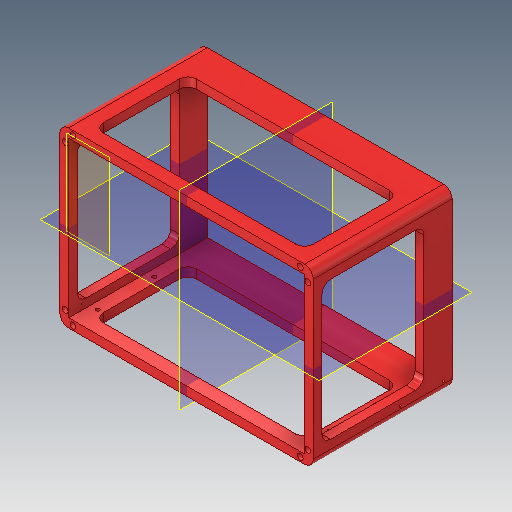
# Autodesk Inventor part: 05_Omniscope_base_v1
Saved by Autodesk Inventor 2019.4 (Build 234330000, 330)
## iProperties
Created: 2021-09-23
Part Number: 05_Omniscope_base_v1
Material: Generisch
Document SubType Name: Modeling
Designer: Muriel
Density: 1 g/cm^3
Appearance: Light Red
Author: Muriel
Autodesk Inventor part; units mm, degrees
ref_plane "Arbeitsebene1" through (0, 0, 0) normal (0, 0, 1) x (1, 0, 0)
sketch "Skizze1" plane through (0, 0, 0) normal (0, 0, 1) x (1, 0, 0)
  arc A0 (4.5124, -17.9) -> (2.1124, -17.9) centre (3.3124, -16.3) ccw construction
  line L0 (4.5124, -17.9) -> (5.3124, -17.9) construction
  line L1 (5.3124, -17.9) -> (6.3124, -16.9) construction
  line L2 (6.3124, -16.9) -> (6.3124, 16.9) construction
  line L3 (6.3124, 16.9) -> (5.3124, 17.9) construction
  line L4 (5.3124, 17.9) -> (4.5124, 17.9) construction
  arc A1 (2.1124, 17.9) -> (4.5124, 17.9) centre (3.3124, 16.3) ccw construction
  line L5 (2.1124, 17.9) -> (-7.2876, 17.9) construction
  arc A2 (-9.6876, 17.9) -> (-7.2876, 17.9) centre (-8.4876, 16.3) ccw construction
  line L6 (-9.6876, 17.9) -> (-10.4876, 17.9) construction
  line L7 (-10.4876, 17.9) -> (-11.4876, 16.9) construction
  line L8 (-11.4876, 16.9) -> (-11.4876, -16.9) construction
  line L9 (-11.4876, -16.9) -> (-10.4876, -17.9) construction
  line L10 (-10.4876, -17.9) -> (-9.6876, -17.9) construction
  arc A3 (-7.2876, -17.9) -> (-9.6876, -17.9) centre (-8.4876, -16.3) ccw construction
  line L11 (-7.2876, -17.9) -> (2.1124, -17.9) construction
  line L12 (1.5472, -2.3689) -> (1.5472, -5.8689) construction
  line L13 (1.5472, -5.8689) -> (1.0253, -5.8689) construction
  line L14 (1.0253, -5.8689) -> (-0.5233, -2.8511) construction
  line L15 (-0.5233, -2.8511) -> (-0.5233, -5.8689) construction
  line L16 (-0.5233, -5.8689) -> (-0.9572, -5.8689) construction
  line L17 (-0.9572, -5.8689) -> (-0.9572, -2.3689) construction
  line L18 (-0.9572, -2.3689) -> (-0.2964, -2.3689) construction
  line L19 (-0.2964, -2.3689) -> (1.1133, -5.14) construction
  line L20 (1.1133, -5.14) -> (1.1133, -2.3689) construction
  line L21 (1.1133, -2.3689) -> (1.5472, -2.3689) construction
  line L22 (4.5026, -1.0603) -> (4.5026, -1.4177) construction
  line L23 (4.5026, -1.4177) -> (2.7952, -1.4177) construction
  line L24 (2.7952, -1.4177) -> (2.7952, -1.0603) construction
  line L25 (2.7952, -1.0603) -> (3.4305, -1.0603) construction
  line L26 (3.4305, -1.0603) -> (3.4305, 1.2853) construction
  line L27 (3.4305, 1.2853) -> (2.7952, 1.2853) construction
  line L28 (2.7952, 1.2853) -> (2.7952, 1.6058) construction
  spline S0 degree 2 poles (2.7952, 1.6058) (3.1554, 1.6058) (3.4957, 1.81) (3.5184, 2.0937) knots 0 0 0 1 2 2 2 construction
  line L29 (3.5184, 2.0937) -> (3.8815, 2.0937) construction
  line L30 (3.8815, 2.0937) -> (3.8815, -1.0603) construction
  line L31 (3.8815, -1.0603) -> (4.5026, -1.0603) construction
  line L32 (4.5665, 6.9442) -> (5.0401, 6.9442) construction
  line L33 (5.0401, 6.9442) -> (3.8347, 3.4442) construction
  line L34 (3.8347, 3.4442) -> (3.3327, 3.4442) construction
  line L35 (3.3327, 3.4442) -> (2.1272, 6.9442) construction
  line L36 (2.1272, 6.9442) -> (2.6264, 6.9442) construction
  line L37 (2.6264, 6.9442) -> (3.5964, 4.037) construction
  line L38 (3.5964, 4.037) -> (4.5665, 6.9442) construction
  spline S1 degree 2 poles (1.5373, 5.4012) (1.7103, 5.2708) (1.8975, 4.8737) (1.8975, 4.556) knots 0 0 0 1 2 2 2 construction
  spline S2 degree 2 poles (1.8975, 4.556) (1.8975, 4.3036) (1.7358, 3.8725) (1.5883, 3.7136) knots 0 0 0 1 2 2 2 construction
  spline S3 degree 2 poles (1.5883, 3.7136) (1.4408, 3.5548) (1.0012, 3.3704) (0.7289, 3.3704) knots 0 0 0 1 2 2 2 construction
  spline S4 degree 2 poles (0.7289, 3.3704) (0.4793, 3.3704) (-0.0085, 3.4811) (-0.1872, 3.569) knots 0 0 0 1 2 2 2 construction
  line L39 (-0.1872, 3.569) -> (-0.1872, 4.0653) construction
  line L40 (-0.1872, 4.0653) -> (-0.1532, 4.0653) construction
  spline S5 degree 2 poles (-0.1532, 4.0653) (-0.0993, 4.0256) (0.1021, 3.9235) (0.2241, 3.8781) knots 0 0 0 1 2 2 2 construction
  spline S6 degree 2 poles (0.2241, 3.8781) (0.363, 3.8299) (0.5928, 3.776) (0.7374, 3.776) knots 0 0 0 1 2 2 2 construction
  spline S7 degree 2 poles (0.7374, 3.776) (0.8793, 3.776) (1.1459, 3.8781) (1.2423, 3.9888) knots 0 0 0 1 2 2 2 construction
  spline S8 degree 2 poles (1.2423, 3.9888) (1.3302, 4.0937) (1.421, 4.3717) (1.421, 4.5589) knots 0 0 0 1 2 2 2 construction
  spline S9 degree 2 poles (1.421, 4.5589) (1.421, 4.7461) (1.3189, 4.9843) (1.2224, 5.0637) knots 0 0 0 1 2 2 2 construction
  spline S10 degree 2 poles (1.2224, 5.0637) (1.1232, 5.1516) (0.8282, 5.2254) (0.6495, 5.2254) knots 0 0 0 1 2 2 2 construction
  spline S11 degree 2 poles (0.6495, 5.2254) (0.4566, 5.2254) (0.0737, 5.1658) (-0.0425, 5.1403) knots 0 0 0 1 2 2 2 construction
  line L41 (-0.0425, 5.1403) -> (-0.0425, 6.9442) construction
  line L42 (-0.0425, 6.9442) -> (1.8776, 6.9442) construction
  line L43 (1.8776, 6.9442) -> (1.8776, 6.5329) construction
  line L44 (1.8776, 6.5329) -> (0.4084, 6.5329) construction
  line L45 (0.4084, 6.5329) -> (0.4084, 5.5998) construction
  spline S12 degree 2 poles (0.4084, 5.5998) (0.4935, 5.6111) (0.658, 5.6196) (0.7261, 5.6196) knots 0 0 0 1 2 2 2 construction
  spline S13 degree 2 poles (0.7261, 5.6196) (0.9955, 5.6196) (1.3671, 5.5317) (1.5373, 5.4012) knots 0 0 0 1 2 2 2 construction
  line L46 (1.0905, -1.4177) -> (0.6254, -1.4177) construction
  line L47 (0.6254, -1.4177) -> (0.6254, 1.6682) construction
  line L48 (0.6254, 1.6682) -> (-0.5488, 1.6682) construction
  line L49 (-0.5488, 1.6682) -> (-0.5488, 2.0823) construction
  line L50 (-0.5488, 2.0823) -> (2.2648, 2.0823) construction
  line L51 (2.2648, 2.0823) -> (2.2648, 1.6682) construction
  line L52 (2.2648, 1.6682) -> (1.0905, 1.6682) construction
  line L53 (1.0905, 1.6682) -> (1.0905, -1.4177) construction
  spline S14 degree 2 poles (-2.0577, -5.8349) (-2.2307, -5.886) (-2.5087, -5.937) (-2.7044, -5.937) knots 0 0 0 1 2 2 2 construction
  spline S15 degree 2 poles (-2.7044, -5.937) (-3.076, -5.937) (-3.6914, -5.7101) (-3.9127, -5.4804) knots 0 0 0 1 2 2 2 construction
  spline S16 degree 2 poles (-3.9127, -5.4804) (-4.1339, -5.2478) (-4.3693, -4.5614) (-4.3693, -4.1161) knots 0 0 0 1 2 2 2 construction
  spline S17 degree 2 poles (-4.3693, -4.1161) (-4.3693, -3.6935) (-4.1311, -3.0241) (-3.9098, -2.7859) knots 0 0 0 1 2 2 2 construction
  spline S18 degree 2 poles (-3.9098, -2.7859) (-3.6971, -2.5561) (-3.0731, -2.3065) (-2.7016, -2.3065) knots 0 0 0 1 2 2 2 construction
  spline S19 degree 2 poles (-2.7016, -2.3065) (-2.5229, -2.3065) (-2.1995, -2.3576) (-2.052, -2.403) knots 0 0 0 1 2 2 2 construction
  spline S20 degree 2 poles (-2.052, -2.403) (-1.9329, -2.437) (-1.6436, -2.5618) (-1.5557, -2.6072) knots 0 0 0 1 2 2 2 construction
  line L54 (-1.5557, -2.6072) -> (-1.5557, -3.1688) construction
  line L55 (-1.5557, -3.1688) -> (-1.5954, -3.1688) construction
  spline S21 degree 2 poles (-1.5954, -3.1688) (-1.6833, -3.0922) (-1.8677, -2.9532) (-2.0379, -2.8738) knots 0 0 0 1 2 2 2 construction
  spline S22 degree 2 poles (-2.0379, -2.8738) (-2.1797, -2.8029) (-2.5456, -2.7093) (-2.7554, -2.7093) knots 0 0 0 1 2 2 2 construction
  spline S23 degree 2 poles (-2.7554, -2.7093) (-3.2603, -2.7093) (-3.8843, -3.4694) (-3.8843, -4.1019) knots 0 0 0 1 2 2 2 construction
  spline S24 degree 2 poles (-3.8843, -4.1019) (-3.8843, -4.4536) (-3.7198, -4.9812) (-3.5638, -5.1627) knots 0 0 0 1 2 2 2 construction
  spline S25 degree 2 poles (-3.5638, -5.1627) (-3.4135, -5.3442) (-2.988, -5.5343) (-2.7214, -5.5343) knots 0 0 0 1 2 2 2 construction
  spline S26 degree 2 poles (-2.7214, -5.5343) (-2.5257, -5.5343) (-2.1343, -5.4775) (-2.001, -5.4208) knots 0 0 0 1 2 2 2 construction
  line L56 (-2.001, -5.4208) -> (-2.001, -4.516) construction
  line L57 (-2.001, -4.516) -> (-2.8122, -4.516) construction
  line L58 (-2.8122, -4.516) -> (-2.8122, -4.1076) construction
  line L59 (-2.8122, -4.1076) -> (-1.5415, -4.1076) construction
  line L60 (-1.5415, -4.1076) -> (-1.5415, -5.6364) construction
  spline S27 degree 2 poles (-1.5415, -5.6364) (-1.6294, -5.6761) (-1.9301, -5.798) (-2.0577, -5.8349) knots 0 0 0 1 2 2 2 construction
  spline S28 degree 2 poles (4.307, -2.6469) (4.6445, -2.871) (5.016, -3.6112) (5.016, -4.1218) knots 0 0 0 1 2 2 2 construction
  spline S29 degree 2 poles (5.016, -4.1218) (5.016, -4.6011) (4.6275, -5.3726) (4.3013, -5.5881) knots 0 0 0 1 2 2 2 construction
  spline S30 degree 2 poles (4.3013, -5.5881) (4.0347, -5.7555) (3.4873, -5.8689) (3.0618, -5.8689) knots 0 0 0 1 2 2 2 construction
  line L61 (3.0618, -5.8689) -> (2.2563, -5.8689) construction
  line L62 (2.2563, -5.8689) -> (2.2563, -2.3689) construction
  line L63 (2.2563, -2.3689) -> (3.0533, -2.3689) construction
  spline S31 degree 2 poles (3.0533, -2.3689) (3.5468, -2.3689) (4.1084, -2.5164) (4.307, -2.6469) knots 0 0 0 1 2 2 2 construction
  arc A4 (4.5124, -53.9) -> (2.1124, -53.9) centre (3.3124, -52.3) ccw construction
  line L64 (4.5124, -53.9) -> (5.3124, -53.9) construction
  line L65 (5.3124, -53.9) -> (6.3124, -52.9) construction
  line L66 (6.3124, -52.9) -> (6.3124, -19.1) construction
  line L67 (6.3124, -19.1) -> (5.3124, -18.1) construction
  line L68 (5.3124, -18.1) -> (4.5124, -18.1) construction
  arc A5 (2.1124, -18.1) -> (4.5124, -18.1) centre (3.3124, -19.7) ccw construction
  line L69 (2.1124, -18.1) -> (-7.2876, -18.1) construction
  arc A6 (-9.6876, -18.1) -> (-7.2876, -18.1) centre (-8.4876, -19.7) ccw construction
  line L70 (-9.6876, -18.1) -> (-10.4876, -18.1) construction
  line L71 (-10.4876, -18.1) -> (-11.4876, -19.1) construction
  line L72 (-11.4876, -19.1) -> (-11.4876, -52.9) construction
  line L73 (-11.4876, -52.9) -> (-10.4876, -53.9) construction
  line L74 (-10.4876, -53.9) -> (-9.6876, -53.9) construction
  arc A7 (-7.2876, -53.9) -> (-9.6876, -53.9) centre (-8.4876, -52.3) ccw construction
  line L75 (-7.2876, -53.9) -> (2.1124, -53.9) construction
  line L76 (1.5472, -38.3689) -> (1.5472, -41.8689) construction
  line L77 (1.5472, -41.8689) -> (1.0253, -41.8689) construction
  line L78 (1.0253, -41.8689) -> (-0.5233, -38.8511) construction
  line L79 (-0.5233, -38.8511) -> (-0.5233, -41.8689) construction
  line L80 (-0.5233, -41.8689) -> (-0.9572, -41.8689) construction
  line L81 (-0.9572, -41.8689) -> (-0.9572, -38.3689) construction
  line L82 (-0.9572, -38.3689) -> (-0.2964, -38.3689) construction
  line L83 (-0.2964, -38.3689) -> (1.1133, -41.14) construction
  line L84 (1.1133, -41.14) -> (1.1133, -38.3689) construction
  line L85 (1.1133, -38.3689) -> (1.5472, -38.3689) construction
  line L86 (4.5026, -37.0603) -> (4.5026, -37.4177) construction
  line L87 (4.5026, -37.4177) -> (2.7952, -37.4177) construction
  line L88 (2.7952, -37.4177) -> (2.7952, -37.0603) construction
  line L89 (2.7952, -37.0603) -> (3.4305, -37.0603) construction
  line L90 (3.4305, -37.0603) -> (3.4305, -34.7147) construction
  line L91 (3.4305, -34.7147) -> (2.7952, -34.7147) construction
  line L92 (2.7952, -34.7147) -> (2.7952, -34.3942) construction
  spline S32 degree 2 poles (2.7952, -34.3942) (3.1554, -34.3942) (3.4957, -34.19) (3.5184, -33.9063) knots 0 0 0 1 2 2 2 construction
  line L93 (3.5184, -33.9063) -> (3.8815, -33.9063) construction
  line L94 (3.8815, -33.9063) -> (3.8815, -37.0603) construction
  line L95 (3.8815, -37.0603) -> (4.5026, -37.0603) construction
  line L96 (4.5665, -29.0558) -> (5.0401, -29.0558) construction
  line L97 (5.0401, -29.0558) -> (3.8347, -32.5558) construction
  line L98 (3.8347, -32.5558) -> (3.3327, -32.5558) construction
  line L99 (3.3327, -32.5558) -> (2.1272, -29.0558) construction
  line L100 (2.1272, -29.0558) -> (2.6264, -29.0558) construction
  line L101 (2.6264, -29.0558) -> (3.5964, -31.963) construction
  line L102 (3.5964, -31.963) -> (4.5665, -29.0558) construction
  spline S33 degree 2 poles (1.5373, -30.5988) (1.7103, -30.7292) (1.8975, -31.1263) (1.8975, -31.444) knots 0 0 0 1 2 2 2 construction
  spline S34 degree 2 poles (1.8975, -31.444) (1.8975, -31.6964) (1.7358, -32.1275) (1.5883, -32.2864) knots 0 0 0 1 2 2 2 construction
  spline S35 degree 2 poles (1.5883, -32.2864) (1.4408, -32.4452) (1.0012, -32.6296) (0.7289, -32.6296) knots 0 0 0 1 2 2 2 construction
  spline S36 degree 2 poles (0.7289, -32.6296) (0.4793, -32.6296) (-0.0085, -32.5189) (-0.1872, -32.431) knots 0 0 0 1 2 2 2 construction
  line L103 (-0.1872, -32.431) -> (-0.1872, -31.9347) construction
  line L104 (-0.1872, -31.9347) -> (-0.1532, -31.9347) construction
  spline S37 degree 2 poles (-0.1532, -31.9347) (-0.0993, -31.9744) (0.1021, -32.0765) (0.2241, -32.1219) knots 0 0 0 1 2 2 2 construction
  spline S38 degree 2 poles (0.2241, -32.1219) (0.363, -32.1701) (0.5928, -32.224) (0.7374, -32.224) knots 0 0 0 1 2 2 2 construction
  spline S39 degree 2 poles (0.7374, -32.224) (0.8793, -32.224) (1.1459, -32.1219) (1.2423, -32.0112) knots 0 0 0 1 2 2 2 construction
  spline S40 degree 2 poles (1.2423, -32.0112) (1.3302, -31.9063) (1.421, -31.6283) (1.421, -31.4411) knots 0 0 0 1 2 2 2 construction
  spline S41 degree 2 poles (1.421, -31.4411) (1.421, -31.2539) (1.3189, -31.0157) (1.2224, -30.9363) knots 0 0 0 1 2 2 2 construction
  spline S42 degree 2 poles (1.2224, -30.9363) (1.1232, -30.8484) (0.8282, -30.7746) (0.6495, -30.7746) knots 0 0 0 1 2 2 2 construction
  spline S43 degree 2 poles (0.6495, -30.7746) (0.4566, -30.7746) (0.0737, -30.8342) (-0.0425, -30.8597) knots 0 0 0 1 2 2 2 construction
  line L105 (-0.0425, -30.8597) -> (-0.0425, -29.0558) construction
  line L106 (-0.0425, -29.0558) -> (1.8776, -29.0558) construction
  line L107 (1.8776, -29.0558) -> (1.8776, -29.4671) construction
  line L108 (1.8776, -29.4671) -> (0.4084, -29.4671) construction
  line L109 (0.4084, -29.4671) -> (0.4084, -30.4002) construction
  spline S44 degree 2 poles (0.4084, -30.4002) (0.4935, -30.3889) (0.658, -30.3804) (0.7261, -30.3804) knots 0 0 0 1 2 2 2 construction
  spline S45 degree 2 poles (0.7261, -30.3804) (0.9955, -30.3804) (1.3671, -30.4683) (1.5373, -30.5988) knots 0 0 0 1 2 2 2 construction
  line L110 (1.0905, -37.4177) -> (0.6254, -37.4177) construction
  line L111 (0.6254, -37.4177) -> (0.6254, -34.3318) construction
  line L112 (0.6254, -34.3318) -> (-0.5488, -34.3318) construction
  line L113 (-0.5488, -34.3318) -> (-0.5488, -33.9177) construction
  line L114 (-0.5488, -33.9177) -> (2.2648, -33.9177) construction
  line L115 (2.2648, -33.9177) -> (2.2648, -34.3318) construction
  line L116 (2.2648, -34.3318) -> (1.0905, -34.3318) construction
  line L117 (1.0905, -34.3318) -> (1.0905, -37.4177) construction
  spline S46 degree 2 poles (-2.0577, -41.8349) (-2.2307, -41.886) (-2.5087, -41.937) (-2.7044, -41.937) knots 0 0 0 1 2 2 2 construction
  spline S47 degree 2 poles (-2.7044, -41.937) (-3.076, -41.937) (-3.6914, -41.7101) (-3.9127, -41.4804) knots 0 0 0 1 2 2 2 construction
  spline S48 degree 2 poles (-3.9127, -41.4804) (-4.1339, -41.2478) (-4.3693, -40.5614) (-4.3693, -40.1161) knots 0 0 0 1 2 2 2 construction
  spline S49 degree 2 poles (-4.3693, -40.1161) (-4.3693, -39.6935) (-4.1311, -39.0241) (-3.9098, -38.7859) knots 0 0 0 1 2 2 2 construction
  spline S50 degree 2 poles (-3.9098, -38.7859) (-3.6971, -38.5561) (-3.0731, -38.3065) (-2.7016, -38.3065) knots 0 0 0 1 2 2 2 construction
  spline S51 degree 2 poles (-2.7016, -38.3065) (-2.5229, -38.3065) (-2.1995, -38.3576) (-2.052, -38.403) knots 0 0 0 1 2 2 2 construction
  spline S52 degree 2 poles (-2.052, -38.403) (-1.9329, -38.437) (-1.6436, -38.5618) (-1.5557, -38.6072) knots 0 0 0 1 2 2 2 construction
  line L118 (-1.5557, -38.6072) -> (-1.5557, -39.1688) construction
  line L119 (-1.5557, -39.1688) -> (-1.5954, -39.1688) construction
  spline S53 degree 2 poles (-1.5954, -39.1688) (-1.6833, -39.0922) (-1.8677, -38.9532) (-2.0379, -38.8738) knots 0 0 0 1 2 2 2 construction
  spline S54 degree 2 poles (-2.0379, -38.8738) (-2.1797, -38.8029) (-2.5456, -38.7093) (-2.7554, -38.7093) knots 0 0 0 1 2 2 2 construction
  spline S55 degree 2 poles (-2.7554, -38.7093) (-3.2603, -38.7093) (-3.8843, -39.4694) (-3.8843, -40.1019) knots 0 0 0 1 2 2 2 construction
  spline S56 degree 2 poles (-3.8843, -40.1019) (-3.8843, -40.4536) (-3.7198, -40.9812) (-3.5638, -41.1627) knots 0 0 0 1 2 2 2 construction
  spline S57 degree 2 poles (-3.5638, -41.1627) (-3.4135, -41.3442) (-2.988, -41.5343) (-2.7214, -41.5343) knots 0 0 0 1 2 2 2 construction
  spline S58 degree 2 poles (-2.7214, -41.5343) (-2.5257, -41.5343) (-2.1343, -41.4775) (-2.001, -41.4208) knots 0 0 0 1 2 2 2 construction
  line L120 (-2.001, -41.4208) -> (-2.001, -40.516) construction
  line L121 (-2.001, -40.516) -> (-2.8122, -40.516) construction
  line L122 (-2.8122, -40.516) -> (-2.8122, -40.1076) construction
  line L123 (-2.8122, -40.1076) -> (-1.5415, -40.1076) construction
  line L124 (-1.5415, -40.1076) -> (-1.5415, -41.6364) construction
  spline S59 degree 2 poles (-1.5415, -41.6364) (-1.6294, -41.6761) (-1.9301, -41.798) (-2.0577, -41.8349) knots 0 0 0 1 2 2 2 construction
  spline S60 degree 2 poles (4.307, -38.6469) (4.6445, -38.871) (5.016, -39.6112) (5.016, -40.1218) knots 0 0 0 1 2 2 2 construction
  spline S61 degree 2 poles (5.016, -40.1218) (5.016, -40.6011) (4.6275, -41.3726) (4.3013, -41.5881) knots 0 0 0 1 2 2 2 construction
  spline S62 degree 2 poles (4.3013, -41.5881) (4.0347, -41.7555) (3.4873, -41.8689) (3.0618, -41.8689) knots 0 0 0 1 2 2 2 construction
  line L125 (3.0618, -41.8689) -> (2.2563, -41.8689) construction
  line L126 (2.2563, -41.8689) -> (2.2563, -38.3689) construction
  line L127 (2.2563, -38.3689) -> (3.0533, -38.3689) construction
  spline S63 degree 2 poles (3.0533, -38.3689) (3.5468, -38.3689) (4.1084, -38.5164) (4.307, -38.6469) knots 0 0 0 1 2 2 2 construction
  arc A8 (94.5124, -53.9) -> (92.1124, -53.9) centre (93.3124, -52.3) ccw construction
  line L128 (94.5124, -53.9) -> (95.3124, -53.9) construction
  line L129 (95.3124, -53.9) -> (96.3124, -52.9) construction
  line L130 (96.3124, -52.9) -> (96.3124, -19.1) construction
  line L131 (96.3124, -19.1) -> (95.3124, -18.1) construction
  line L132 (95.3124, -18.1) -> (94.5124, -18.1) construction
  arc A9 (92.1124, -18.1) -> (94.5124, -18.1) centre (93.3124, -19.7) ccw construction
  line L133 (92.1124, -18.1) -> (82.7124, -18.1) construction
  arc A10 (80.3124, -18.1) -> (82.7124, -18.1) centre (81.5124, -19.7) ccw construction
  line L134 (80.3124, -18.1) -> (79.5124, -18.1) construction
  line L135 (79.5124, -18.1) -> (78.5124, -19.1) construction
  line L136 (78.5124, -19.1) -> (78.5124, -52.9) construction
  line L137 (78.5124, -52.9) -> (79.5124, -53.9) construction
  line L138 (79.5124, -53.9) -> (80.3124, -53.9) construction
  arc A11 (82.7124, -53.9) -> (80.3124, -53.9) centre (81.5124, -52.3) ccw construction
  line L139 (82.7124, -53.9) -> (92.1124, -53.9) construction
  line L140 (91.5472, -38.3689) -> (91.5472, -41.8689) construction
  line L141 (91.5472, -41.8689) -> (91.0253, -41.8689) construction
  line L142 (91.0253, -41.8689) -> (89.4767, -38.8511) construction
  line L143 (89.4767, -38.8511) -> (89.4767, -41.8689) construction
  line L144 (89.4767, -41.8689) -> (89.0428, -41.8689) construction
  line L145 (89.0428, -41.8689) -> (89.0428, -38.3689) construction
  line L146 (89.0428, -38.3689) -> (89.7036, -38.3689) construction
  line L147 (89.7036, -38.3689) -> (91.1133, -41.14) construction
  line L148 (91.1133, -41.14) -> (91.1133, -38.3689) construction
  line L149 (91.1133, -38.3689) -> (91.5472, -38.3689) construction
  line L150 (94.5026, -37.0603) -> (94.5026, -37.4177) construction
  line L151 (94.5026, -37.4177) -> (92.7952, -37.4177) construction
  line L152 (92.7952, -37.4177) -> (92.7952, -37.0603) construction
  line L153 (92.7952, -37.0603) -> (93.4305, -37.0603) construction
  line L154 (93.4305, -37.0603) -> (93.4305, -34.7147) construction
  line L155 (93.4305, -34.7147) -> (92.7952, -34.7147) construction
  line L156 (92.7952, -34.7147) -> (92.7952, -34.3942) construction
  spline S64 degree 2 poles (92.7952, -34.3942) (93.1554, -34.3942) (93.4957, -34.19) (93.5184, -33.9063) knots 0 0 0 1 2 2 2 construction
  line L157 (93.5184, -33.9063) -> (93.8815, -33.9063) construction
  line L158 (93.8815, -33.9063) -> (93.8815, -37.0603) construction
  line L159 (93.8815, -37.0603) -> (94.5026, -37.0603) construction
  line L160 (94.5665, -29.0558) -> (95.0401, -29.0558) construction
  line L161 (95.0401, -29.0558) -> (93.8347, -32.5558) construction
  line L162 (93.8347, -32.5558) -> (93.3327, -32.5558) construction
  line L163 (93.3327, -32.5558) -> (92.1272, -29.0558) construction
  line L164 (92.1272, -29.0558) -> (92.6264, -29.0558) construction
  line L165 (92.6264, -29.0558) -> (93.5964, -31.963) construction
  line L166 (93.5964, -31.963) -> (94.5665, -29.0558) construction
  spline S65 degree 2 poles (91.5373, -30.5988) (91.7103, -30.7292) (91.8975, -31.1263) (91.8975, -31.444) knots 0 0 0 1 2 2 2 construction
  spline S66 degree 2 poles (91.8975, -31.444) (91.8975, -31.6964) (91.7358, -32.1275) (91.5883, -32.2864) knots 0 0 0 1 2 2 2 construction
  spline S67 degree 2 poles (91.5883, -32.2864) (91.4408, -32.4452) (91.0012, -32.6296) (90.7289, -32.6296) knots 0 0 0 1 2 2 2 construction
  spline S68 degree 2 poles (90.7289, -32.6296) (90.4793, -32.6296) (89.9915, -32.5189) (89.8128, -32.431) knots 0 0 0 1 2 2 2 construction
  line L167 (89.8128, -32.431) -> (89.8128, -31.9347) construction
  line L168 (89.8128, -31.9347) -> (89.8468, -31.9347) construction
  spline S69 degree 2 poles (89.8468, -31.9347) (89.9007, -31.9744) (90.1021, -32.0765) (90.2241, -32.1219) knots 0 0 0 1 2 2 2 construction
  spline S70 degree 2 poles (90.2241, -32.1219) (90.363, -32.1701) (90.5928, -32.224) (90.7374, -32.224) knots 0 0 0 1 2 2 2 construction
  spline S71 degree 2 poles (90.7374, -32.224) (90.8793, -32.224) (91.1459, -32.1219) (91.2423, -32.0112) knots 0 0 0 1 2 2 2 construction
  spline S72 degree 2 poles (91.2423, -32.0112) (91.3302, -31.9063) (91.421, -31.6283) (91.421, -31.4411) knots 0 0 0 1 2 2 2 construction
  spline S73 degree 2 poles (91.421, -31.4411) (91.421, -31.2539) (91.3189, -31.0157) (91.2224, -30.9363) knots 0 0 0 1 2 2 2 construction
  spline S74 degree 2 poles (91.2224, -30.9363) (91.1232, -30.8484) (90.8282, -30.7746) (90.6495, -30.7746) knots 0 0 0 1 2 2 2 construction
  spline S75 degree 2 poles (90.6495, -30.7746) (90.4566, -30.7746) (90.0737, -30.8342) (89.9575, -30.8597) knots 0 0 0 1 2 2 2 construction
  line L169 (89.9575, -30.8597) -> (89.9575, -29.0558) construction
  line L170 (89.9575, -29.0558) -> (91.8776, -29.0558) construction
  line L171 (91.8776, -29.0558) -> (91.8776, -29.4671) construction
  line L172 (91.8776, -29.4671) -> (90.4084, -29.4671) construction
  line L173 (90.4084, -29.4671) -> (90.4084, -30.4002) construction
  spline S76 degree 2 poles (90.4084, -30.4002) (90.4935, -30.3889) (90.658, -30.3804) (90.7261, -30.3804) knots 0 0 0 1 2 2 2 construction
  spline S77 degree 2 poles (90.7261, -30.3804) (90.9955, -30.3804) (91.3671, -30.4683) (91.5373, -30.5988) knots 0 0 0 1 2 2 2 construction
  line L174 (91.0905, -37.4177) -> (90.6254, -37.4177) construction
  line L175 (90.6254, -37.4177) -> (90.6254, -34.3318) construction
  line L176 (90.6254, -34.3318) -> (89.4512, -34.3318) construction
  line L177 (89.4512, -34.3318) -> (89.4512, -33.9177) construction
  line L178 (89.4512, -33.9177) -> (92.2648, -33.9177) construction
  line L179 (92.2648, -33.9177) -> (92.2648, -34.3318) construction
  line L180 (92.2648, -34.3318) -> (91.0905, -34.3318) construction
  line L181 (91.0905, -34.3318) -> (91.0905, -37.4177) construction
  spline S78 degree 2 poles (87.9423, -41.8349) (87.7693, -41.886) (87.4913, -41.937) (87.2956, -41.937) knots 0 0 0 1 2 2 2 construction
  spline S79 degree 2 poles (87.2956, -41.937) (86.924, -41.937) (86.3086, -41.7101) (86.0873, -41.4804) knots 0 0 0 1 2 2 2 construction
  spline S80 degree 2 poles (86.0873, -41.4804) (85.8661, -41.2478) (85.6307, -40.5614) (85.6307, -40.1161) knots 0 0 0 1 2 2 2 construction
  spline S81 degree 2 poles (85.6307, -40.1161) (85.6307, -39.6935) (85.8689, -39.0241) (86.0902, -38.7859) knots 0 0 0 1 2 2 2 construction
  spline S82 degree 2 poles (86.0902, -38.7859) (86.3029, -38.5561) (86.9269, -38.3065) (87.2984, -38.3065) knots 0 0 0 1 2 2 2 construction
  spline S83 degree 2 poles (87.2984, -38.3065) (87.4771, -38.3065) (87.8005, -38.3576) (87.948, -38.403) knots 0 0 0 1 2 2 2 construction
  spline S84 degree 2 poles (87.948, -38.403) (88.0671, -38.437) (88.3564, -38.5618) (88.4443, -38.6072) knots 0 0 0 1 2 2 2 construction
  line L182 (88.4443, -38.6072) -> (88.4443, -39.1688) construction
  line L183 (88.4443, -39.1688) -> (88.4046, -39.1688) construction
  spline S85 degree 2 poles (88.4046, -39.1688) (88.3167, -39.0922) (88.1323, -38.9532) (87.9621, -38.8738) knots 0 0 0 1 2 2 2 construction
  spline S86 degree 2 poles (87.9621, -38.8738) (87.8203, -38.8029) (87.4544, -38.7093) (87.2446, -38.7093) knots 0 0 0 1 2 2 2 construction
  spline S87 degree 2 poles (87.2446, -38.7093) (86.7397, -38.7093) (86.1157, -39.4694) (86.1157, -40.1019) knots 0 0 0 1 2 2 2 construction
  spline S88 degree 2 poles (86.1157, -40.1019) (86.1157, -40.4536) (86.2802, -40.9812) (86.4362, -41.1627) knots 0 0 0 1 2 2 2 construction
  spline S89 degree 2 poles (86.4362, -41.1627) (86.5865, -41.3442) (87.012, -41.5343) (87.2786, -41.5343) knots 0 0 0 1 2 2 2 construction
  spline S90 degree 2 poles (87.2786, -41.5343) (87.4743, -41.5343) (87.8657, -41.4775) (87.999, -41.4208) knots 0 0 0 1 2 2 2 construction
  line L184 (87.999, -41.4208) -> (87.999, -40.516) construction
  line L185 (87.999, -40.516) -> (87.1878, -40.516) construction
  line L186 (87.1878, -40.516) -> (87.1878, -40.1076) construction
  line L187 (87.1878, -40.1076) -> (88.4585, -40.1076) construction
  line L188 (88.4585, -40.1076) -> (88.4585, -41.6364) construction
  spline S91 degree 2 poles (88.4585, -41.6364) (88.3706, -41.6761) (88.0699, -41.798) (87.9423, -41.8349) knots 0 0 0 1 2 2 2 construction
  spline S92 degree 2 poles (94.307, -38.6469) (94.6445, -38.871) (95.016, -39.6112) (95.016, -40.1218) knots 0 0 0 1 2 2 2 construction
  spline S93 degree 2 poles (95.016, -40.1218) (95.016, -40.6011) (94.6275, -41.3726) (94.3013, -41.5881) knots 0 0 0 1 2 2 2 construction
  spline S94 degree 2 poles (94.3013, -41.5881) (94.0347, -41.7555) (93.4873, -41.8689) (93.0618, -41.8689) knots 0 0 0 1 2 2 2 construction
  line L189 (93.0618, -41.8689) -> (92.2563, -41.8689) construction
  line L190 (92.2563, -41.8689) -> (92.2563, -38.3689) construction
  line L191 (92.2563, -38.3689) -> (93.0533, -38.3689) construction
  spline S95 degree 2 poles (93.0533, -38.3689) (93.5468, -38.3689) (94.1084, -38.5164) (94.307, -38.6469) knots 0 0 0 1 2 2 2 construction
  arc A12 (94.5124, -17.9) -> (92.1124, -17.9) centre (93.3124, -16.3) ccw construction
  line L192 (94.5124, -17.9) -> (95.3124, -17.9) construction
  line L193 (95.3124, -17.9) -> (96.3124, -16.9) construction
  line L194 (96.3124, -16.9) -> (96.3124, 16.9) construction
  line L195 (96.3124, 16.9) -> (95.3124, 17.9) construction
  line L196 (95.3124, 17.9) -> (94.5124, 17.9) construction
  arc A13 (92.1124, 17.9) -> (94.5124, 17.9) centre (93.3124, 16.3) ccw construction
  line L197 (92.1124, 17.9) -> (82.7124, 17.9) construction
  arc A14 (80.3124, 17.9) -> (82.7124, 17.9) centre (81.5124, 16.3) ccw construction
  line L198 (80.3124, 17.9) -> (79.5124, 17.9) construction
  line L199 (79.5124, 17.9) -> (78.5124, 16.9) construction
  line L200 (78.5124, 16.9) -> (78.5124, -16.9) construction
  line L201 (78.5124, -16.9) -> (79.5124, -17.9) construction
  line L202 (79.5124, -17.9) -> (80.3124, -17.9) construction
  arc A15 (82.7124, -17.9) -> (80.3124, -17.9) centre (81.5124, -16.3) ccw construction
  line L203 (82.7124, -17.9) -> (92.1124, -17.9) construction
  line L204 (91.5472, -2.3689) -> (91.5472, -5.8689) construction
  line L205 (91.5472, -5.8689) -> (91.0253, -5.8689) construction
  line L206 (91.0253, -5.8689) -> (89.4767, -2.8511) construction
  line L207 (89.4767, -2.8511) -> (89.4767, -5.8689) construction
  line L208 (89.4767, -5.8689) -> (89.0428, -5.8689) construction
  line L209 (89.0428, -5.8689) -> (89.0428, -2.3689) construction
  line L210 (89.0428, -2.3689) -> (89.7036, -2.3689) construction
  line L211 (89.7036, -2.3689) -> (91.1133, -5.14) construction
  line L212 (91.1133, -5.14) -> (91.1133, -2.3689) construction
  line L213 (91.1133, -2.3689) -> (91.5472, -2.3689) construction
  line L214 (94.5026, -1.0603) -> (94.5026, -1.4177) construction
  line L215 (94.5026, -1.4177) -> (92.7952, -1.4177) construction
  line L216 (92.7952, -1.4177) -> (92.7952, -1.0603) construction
  line L217 (92.7952, -1.0603) -> (93.4305, -1.0603) construction
  line L218 (93.4305, -1.0603) -> (93.4305, 1.2853) construction
  line L219 (93.4305, 1.2853) -> (92.7952, 1.2853) construction
  line L220 (92.7952, 1.2853) -> (92.7952, 1.6058) construction
  spline S96 degree 2 poles (92.7952, 1.6058) (93.1554, 1.6058) (93.4957, 1.81) (93.5184, 2.0937) knots 0 0 0 1 2 2 2 construction
  line L221 (93.5184, 2.0937) -> (93.8815, 2.0937) construction
  line L222 (93.8815, 2.0937) -> (93.8815, -1.0603) construction
  line L223 (93.8815, -1.0603) -> (94.5026, -1.0603) construction
  line L224 (94.5665, 6.9442) -> (95.0401, 6.9442) construction
  line L225 (95.0401, 6.9442) -> (93.8347, 3.4442) construction
  line L226 (93.8347, 3.4442) -> (93.3327, 3.4442) construction
  line L227 (93.3327, 3.4442) -> (92.1272, 6.9442) construction
  line L228 (92.1272, 6.9442) -> (92.6264, 6.9442) construction
  line L229 (92.6264, 6.9442) -> (93.5964, 4.037) construction
  line L230 (93.5964, 4.037) -> (94.5665, 6.9442) construction
  spline S97 degree 2 poles (91.5373, 5.4012) (91.7103, 5.2708) (91.8975, 4.8737) (91.8975, 4.556) knots 0 0 0 1 2 2 2 construction
  spline S98 degree 2 poles (91.8975, 4.556) (91.8975, 4.3036) (91.7358, 3.8725) (91.5883, 3.7136) knots 0 0 0 1 2 2 2 construction
  spline S99 degree 2 poles (91.5883, 3.7136) (91.4408, 3.5548) (91.0012, 3.3704) (90.7289, 3.3704) knots 0 0 0 1 2 2 2 construction
  spline S100 degree 2 poles (90.7289, 3.3704) (90.4793, 3.3704) (89.9915, 3.4811) (89.8128, 3.569) knots 0 0 0 1 2 2 2 construction
  line L231 (89.8128, 3.569) -> (89.8128, 4.0653) construction
  line L232 (89.8128, 4.0653) -> (89.8468, 4.0653) construction
  spline S101 degree 2 poles (89.8468, 4.0653) (89.9007, 4.0256) (90.1021, 3.9235) (90.2241, 3.8781) knots 0 0 0 1 2 2 2 construction
  spline S102 degree 2 poles (90.2241, 3.8781) (90.363, 3.8299) (90.5928, 3.776) (90.7374, 3.776) knots 0 0 0 1 2 2 2 construction
  spline S103 degree 2 poles (90.7374, 3.776) (90.8793, 3.776) (91.1459, 3.8781) (91.2423, 3.9888) knots 0 0 0 1 2 2 2 construction
  spline S104 degree 2 poles (91.2423, 3.9888) (91.3302, 4.0937) (91.421, 4.3717) (91.421, 4.5589) knots 0 0 0 1 2 2 2 construction
  spline S105 degree 2 poles (91.421, 4.5589) (91.421, 4.7461) (91.3189, 4.9843) (91.2224, 5.0637) knots 0 0 0 1 2 2 2 construction
  spline S106 degree 2 poles (91.2224, 5.0637) (91.1232, 5.1516) (90.8282, 5.2254) (90.6495, 5.2254) knots 0 0 0 1 2 2 2 construction
  spline S107 degree 2 poles (90.6495, 5.2254) (90.4566, 5.2254) (90.0737, 5.1658) (89.9575, 5.1403) knots 0 0 0 1 2 2 2 construction
  line L233 (89.9575, 5.1403) -> (89.9575, 6.9442) construction
  line L234 (89.9575, 6.9442) -> (91.8776, 6.9442) construction
  line L235 (91.8776, 6.9442) -> (91.8776, 6.5329) construction
  line L236 (91.8776, 6.5329) -> (90.4084, 6.5329) construction
  line L237 (90.4084, 6.5329) -> (90.4084, 5.5998) construction
  spline S108 degree 2 poles (90.4084, 5.5998) (90.4935, 5.6111) (90.658, 5.6196) (90.7261, 5.6196) knots 0 0 0 1 2 2 2 construction
  spline S109 degree 2 poles (90.7261, 5.6196) (90.9955, 5.6196) (91.3671, 5.5317) (91.5373, 5.4012) knots 0 0 0 1 2 2 2 construction
  line L238 (91.0905, -1.4177) -> (90.6254, -1.4177) construction
  line L239 (90.6254, -1.4177) -> (90.6254, 1.6682) construction
  line L240 (90.6254, 1.6682) -> (89.4512, 1.6682) construction
  line L241 (89.4512, 1.6682) -> (89.4512, 2.0823) construction
  line L242 (89.4512, 2.0823) -> (92.2648, 2.0823) construction
  line L243 (92.2648, 2.0823) -> (92.2648, 1.6682) construction
  line L244 (92.2648, 1.6682) -> (91.0905, 1.6682) construction
  line L245 (91.0905, 1.6682) -> (91.0905, -1.4177) construction
  spline S110 degree 2 poles (87.9423, -5.8349) (87.7693, -5.886) (87.4913, -5.937) (87.2956, -5.937) knots 0 0 0 1 2 2 2 construction
  spline S111 degree 2 poles (87.2956, -5.937) (86.924, -5.937) (86.3086, -5.7101) (86.0873, -5.4804) knots 0 0 0 1 2 2 2 construction
  spline S112 degree 2 poles (86.0873, -5.4804) (85.8661, -5.2478) (85.6307, -4.5614) (85.6307, -4.1161) knots 0 0 0 1 2 2 2 construction
  spline S113 degree 2 poles (85.6307, -4.1161) (85.6307, -3.6935) (85.8689, -3.0241) (86.0902, -2.7859) knots 0 0 0 1 2 2 2 construction
  spline S114 degree 2 poles (86.0902, -2.7859) (86.3029, -2.5561) (86.9269, -2.3065) (87.2984, -2.3065) knots 0 0 0 1 2 2 2 construction
  spline S115 degree 2 poles (87.2984, -2.3065) (87.4771, -2.3065) (87.8005, -2.3576) (87.948, -2.403) knots 0 0 0 1 2 2 2 construction
  spline S116 degree 2 poles (87.948, -2.403) (88.0671, -2.437) (88.3564, -2.5618) (88.4443, -2.6072) knots 0 0 0 1 2 2 2 construction
  line L246 (88.4443, -2.6072) -> (88.4443, -3.1688) construction
  line L247 (88.4443, -3.1688) -> (88.4046, -3.1688) construction
  spline S117 degree 2 poles (88.4046, -3.1688) (88.3167, -3.0922) (88.1323, -2.9532) (87.9621, -2.8738) knots 0 0 0 1 2 2 2 construction
  spline S118 degree 2 poles (87.9621, -2.8738) (87.8203, -2.8029) (87.4544, -2.7093) (87.2446, -2.7093) knots 0 0 0 1 2 2 2 construction
  spline S119 degree 2 poles (87.2446, -2.7093) (86.7397, -2.7093) (86.1157, -3.4694) (86.1157, -4.1019) knots 0 0 0 1 2 2 2 construction
  spline S120 degree 2 poles (86.1157, -4.1019) (86.1157, -4.4536) (86.2802, -4.9812) (86.4362, -5.1627) knots 0 0 0 1 2 2 2 construction
  spline S121 degree 2 poles (86.4362, -5.1627) (86.5865, -5.3442) (87.012, -5.5343) (87.2786, -5.5343) knots 0 0 0 1 2 2 2 construction
  spline S122 degree 2 poles (87.2786, -5.5343) (87.4743, -5.5343) (87.8657, -5.4775) (87.999, -5.4208) knots 0 0 0 1 2 2 2 construction
  line L248 (87.999, -5.4208) -> (87.999, -4.516) construction
  line L249 (87.999, -4.516) -> (87.1878, -4.516) construction
  line L250 (87.1878, -4.516) -> (87.1878, -4.1076) construction
  line L251 (87.1878, -4.1076) -> (88.4585, -4.1076) construction
  line L252 (88.4585, -4.1076) -> (88.4585, -5.6364) construction
  spline S123 degree 2 poles (88.4585, -5.6364) (88.3706, -5.6761) (88.0699, -5.798) (87.9423, -5.8349) knots 0 0 0 1 2 2 2 construction
  spline S124 degree 2 poles (94.307, -2.6469) (94.6445, -2.871) (95.016, -3.6112) (95.016, -4.1218) knots 0 0 0 1 2 2 2 construction
  spline S125 degree 2 poles (95.016, -4.1218) (95.016, -4.6011) (94.6275, -5.3726) (94.3013, -5.5881) knots 0 0 0 1 2 2 2 construction
  spline S126 degree 2 poles (94.3013, -5.5881) (94.0347, -5.7555) (93.4873, -5.8689) (93.0618, -5.8689) knots 0 0 0 1 2 2 2 construction
  line L253 (93.0618, -5.8689) -> (92.2563, -5.8689) construction
  line L254 (92.2563, -5.8689) -> (92.2563, -2.3689) construction
  line L255 (92.2563, -2.3689) -> (93.0533, -2.3689) construction
  spline S127 degree 2 poles (93.0533, -2.3689) (93.5468, -2.3689) (94.1084, -2.5164) (94.307, -2.6469) knots 0 0 0 1 2 2 2 construction
  line L256 (96.9041, 17.6) -> (-11.0959, 17.6)
  line L257 (-11.0959, 17.6) -> (-11.0959, -53.4)
  line L258 (-11.0959, -53.4) -> (96.9041, -53.4)
  line L259 (96.9041, -53.4) -> (96.9041, 17.6)
  line L260 (-15.5959, 22.1) -> (101.4041, 22.1)
  line L261 (101.4041, 22.1) -> (101.4041, -57.9)
  line L262 (101.4041, -57.9) -> (-15.5959, -57.9)
  line L263 (-15.5959, -57.9) -> (-15.5959, 22.1)
  circle A16 centre (93.4124, -25) radius 1.5 projected
  circle A17 centre (81.4124, -47) radius 1.5 projected
  circle A18 centre (81.4124, -25) radius 1.5 projected
  circle A19 centre (93.4124, -47) radius 1.5 projected
  line L264 (82.4461, -29.85) -> (84.9461, -29.85) projected
  line L265 (84.9461, -29.85) -> (84.9461, -42.15) projected
  line L266 (84.9461, -42.15) -> (82.4461, -42.15) projected
  line L267 (82.4461, -42.15) -> (82.4461, -29.85) projected
  circle A20 centre (93.4124, 11) radius 1.5 projected
  circle A21 centre (81.4124, -11) radius 1.5 projected
  circle A22 centre (81.4124, 11) radius 1.5 projected
  circle A23 centre (93.4124, -11) radius 1.5 projected
  line L268 (82.4461, 6.15) -> (84.9461, 6.15) projected
  line L269 (84.9461, 6.15) -> (84.9461, -6.15) projected
  line L270 (84.9461, -6.15) -> (82.4461, -6.15) projected
  line L271 (82.4461, -6.15) -> (82.4461, 6.15) projected
  circle A24 centre (3.4124, 11) radius 1.5 projected
  circle A25 centre (-8.5876, -11) radius 1.5 projected
  circle A26 centre (-8.5876, 11) radius 1.5 projected
  circle A27 centre (3.4124, -11) radius 1.5 projected
  line L272 (-7.5539, 6.15) -> (-5.0539, 6.15) projected
  line L273 (-5.0539, 6.15) -> (-5.0539, -6.15) projected
  line L274 (-5.0539, -6.15) -> (-7.5539, -6.15) projected
  line L275 (-7.5539, -6.15) -> (-7.5539, 6.15) projected
  circle A28 centre (3.4124, -25) radius 1.5 projected
  circle A29 centre (-8.5876, -47) radius 1.5 projected
  circle A30 centre (-8.5876, -25) radius 1.5 projected
  circle A31 centre (3.4124, -47) radius 1.5 projected
  line L276 (-7.5539, -29.85) -> (-5.0539, -29.85) projected
  line L277 (-5.0539, -29.85) -> (-5.0539, -42.15) projected
  line L278 (-5.0539, -42.15) -> (-7.5539, -42.15) projected
  line L279 (-7.5539, -42.15) -> (-7.5539, -29.85) projected
  point P0 (0, 0)
  dimension "d0" = 4.5
  dimension "d53" = 80
  dimension "d54" = 71
  dimension "d55" = 108
  constraints: 16 end point, 4 parallel, 2 perpendicular, 1 horizontal, 3 other
  measures "d0" distance between parallel lines of L256 L260
  measures "d53" distance between parallel lines of L260 L262
  measures "d54" distance between parallel lines of L258 L256
  measures "d55" distance between parallel lines of L257 L259
extrude "Extrusion1" add sketch "Skizze1" along normal blind 4 contours L259 L258 L257 L256 | L260 L261 L262 L263 | A16 | A17 | A18 | A19 | L264 L265 L266 L267 | A20 | A21 | A22 | A23 | L268 L269 L270 L271 | A24 | A25 | A26 | A27 | L272 L273 L274 L275 | A28 | A29 | A30 | A31 | L276 L277 L278 L279
sketch "Skizze3" plane through (0, 0, 0) normal (0, 0, -1) x (-1, 0, 0)
  line L0 (15.5959, 22.1) -> (-101.4041, 22.1) projected
  line L1 (-101.4041, 22.1) -> (-101.4041, -57.9) projected
  line L2 (-101.4041, -57.9) -> (15.5959, -57.9) projected
  line L3 (15.5959, -57.9) -> (15.5959, 22.1) projected
  line L4 (-97.3041, -53.8) -> (-97.3041, 18)
  line L5 (-97.3041, 18) -> (11.4959, 18)
  line L6 (11.4959, 18) -> (11.4959, -53.8)
  line L7 (11.4959, -53.8) -> (-97.3041, -53.8)
  point P0 (0, 0)
  dimension "d16" = 4.1
  dimension "d57" = 71.8
  constraints: 8 end point, 3 other
  measures "d16" distance between parallel lines of L1 L4
  measures "d57" distance between parallel lines of L5 L7
ref_plane "Arbeitsebene2" through (47.4124, 4.95, -60.9) normal (0, 0, -1) x (0, 1, 0)
ref_plane "Arbeitsebene3" through (61.7974, -12.65, -54) normal (0, 0, -1) x (0, 1, 0)
ref_plane "Arbeitsebene4" through (78.5124, -53.9, -59.1) normal (0, 0, -1) x (0, 1, 0)
extrude "Extrusion2" add sketch "Skizze3" along normal blind 64.1
sketch "Skizze4" plane through (-15.5959, -57.9, 4) normal (0, -1, 0) x (1, 0, 0)
  line L0 (117, 0) -> (117, -68.1) projected
  line L1 (0, 0) -> (117, 0) projected
  line L2 (0, 0) -> (0, -68.1) projected
  line L3 (107, -49.1) -> (107, -14)
  line L4 (103, -10) -> (14, -10)
  line L5 (10, -14) -> (10, -49.1)
  line L6 (14, -53.1) -> (103, -53.1)
  arc A0 (103, -53.1) -> (107, -49.1) centre (103, -49.1) ccw
  arc A1 (10, -49.1) -> (14, -53.1) centre (14, -49.1) ccw
  arc A2 (14, -10) -> (10, -14) centre (14, -14) ccw
  arc A3 (107, -14) -> (103, -10) centre (103, -14) ccw
  line L7 (117, -68.1) -> (0, -68.1) projected
  point P0 (15.5959, -4)
  point P1 (107, -53.1)
  point P2 (107, -10)
  point P3 (10, -10)
  point P4 (10, -53.1)
  dimension "d22" = 4
  constraints: 8 end point, 8 point on circle, 8 point on line, 8 tangent, 4 centre point, 3 equal radius, 2 other
  measures "d22" radius of A0
extrude "Extrusion3" cut sketch "Skizze4" against normal through all contours A0 L6 A1 L5 A2 L4 A3 L3
sketch "Skizze5" plane through (-15.5959, -57.9, 4) normal (-1, 0, 0) x (0, 0, 1)
  line L0 (0, 0) -> (-68.1, 0) projected
  line L1 (0, 80) -> (0, 0) projected
  line L2 (-68.1, 80) -> (0, 80) projected
  line L3 (-51.1, 8) -> (-12, 8)
  line L4 (-8, 12) -> (-8, 68)
  line L5 (-12, 72) -> (-51.1, 72)
  line L6 (-55.1, 68) -> (-55.1, 12)
  arc A0 (-55.1, 12) -> (-51.1, 8) centre (-51.1, 12) ccw
  arc A1 (-51.1, 72) -> (-55.1, 68) centre (-51.1, 68) ccw
  arc A2 (-8, 68) -> (-12, 72) centre (-12, 68) ccw
  arc A3 (-12, 8) -> (-8, 12) centre (-12, 12) ccw
  line L7 (-68.1, 0) -> (-68.1, 80) projected
  point P0 (-4, 57.9)
  dimension "d23" = 8
  dimension "d24" = 4
  constraints: 8 end point, 8 point on circle, 8 tangent, 4 centre point, 3 equal radius, 2 other
  measures "d23" distance between parallel lines of L0 L3
  measures "d24" radius of A0
extrude "Extrusion4" cut sketch "Skizze5" against normal through all contours A0 L6 A1 L5 A2 L4 A3 L3
fillet "Rundung1" radius 4 4 edges at (-15.5959, -57.9, -30.05) (-15.5959, 22.1, -30.05) (101.4041, 22.1, -30.05) (101.4041, -57.9, -30.05)
sketch "Skizze6" plane through (96.3476, -57.9, -64.1) normal (0, 0, -1) x (-1, 0, 0)
  line L0 (109.4434, 6.5) -> (-2.5566, 6.5) construction
  line L1 (-2.5566, 6.5) -> (-2.5566, 73.5) construction
  line L2 (-2.5566, 73.5) -> (109.4434, 73.5) construction
  line L3 (109.4434, 73.5) -> (109.4434, 6.5) construction
  line L4 (109.4434, 6.5) -> (-2.5566, 73.5) construction
  line L5 (-2.5566, 6.5) -> (109.4434, 73.5) construction
  line L6 (105.9434, 2) -> (0.9434, 2) construction
  line L7 (0.9434, 2) -> (0.9434, 78) construction
  line L8 (0.9434, 78) -> (105.9434, 78) construction
  line L9 (105.9434, 78) -> (105.9434, 2) construction
  line L10 (105.9434, 2) -> (0.9434, 78) construction
  line L11 (0.9434, 2) -> (105.9434, 78) construction
  line L12 (107.9434, 80) -> (-1.0566, 80) projected
  line L13 (-0.9566, 75.9) -> (107.8434, 75.9) projected
  line L14 (-0.9566, 4.1) -> (-0.9566, 75.9) projected
  line L15 (107.8434, 75.9) -> (107.8434, 4.1) projected
  line L16 (107.8434, 4.1) -> (-0.9566, 4.1) projected
  point P0 (96.3476, 57.9)
  point P1 (53.4434, 40)
  point P2 (53.4434, 40)
  dimension "d28" = 112
  dimension "d29" = 67
  dimension "d30" = 105
  dimension "d31" = 76
  dimension "d56" = 4.1
  dimension "d58" = 108.8
  dimension "d59" = 54.4
  dimension "d60" = 71.8
  dimension "d61" = 35.9
  constraints: 24 end point, 5 midpoint, 4 parallel, 2 horizontal, 2 perpendicular
  measures "d28" distance of L1.end L2.end
  measures "d29" distance of L0.end L1.end
  measures "d30" distance of L7.end L8.end
  measures "d31" distance of L6.end L7.end
  measures "d56" distance between parallel lines of L12 L13
  measures "d58" distance between parallel lines of L14 L15
  measures "d59" distance from line of point (53.443, 40) L15
  measures "d60" distance between parallel lines of L13 L16
  measures "d61" distance from line of point (53.443, 40) L16
hole "Bohrung2" at (-9.5959, 20.1, -64.1) at (-13.0959, 15.6, -64.1) at (-13.0959, -51.4, -64.1) at (-9.5959, -55.9, -64.1) at (95.4041, -55.9, -64.1) at (98.9041, -51.4, -64.1) at (98.9041, 15.6, -64.1) at (95.4041, 20.1, -64.1) direction (0, 0, 1) diameter 2.7 depth 12 tip angle 118
sketch "Skizze7" plane through (0, 0, 4) normal (0, 0, 1) x (1, 0, 0)
  circle A0 centre (-10.1241, 15.5176) radius 1.4
  circle A1 centre (94.8759, 15.5176) radius 1.4
  circle A2 centre (94.8759, -51.4824) radius 1.4
  circle A3 centre (-9.1741, -51.4824) radius 1.4
  circle A4 centre (-13.0959, -51.4) radius 1.35 projected
  circle A5 centre (-9.5959, -55.9) radius 1.35 projected
  circle A6 centre (95.4041, -55.9) radius 1.35 projected
  circle A7 centre (98.9041, -51.4) radius 1.35 projected
  circle A8 centre (98.9041, 15.6) radius 1.35 projected
  circle A9 centre (95.4041, 20.1) radius 1.35 projected
  circle A10 centre (-9.5959, 20.1) radius 1.35 projected
  circle A11 centre (-13.0959, 15.6) radius 1.35 projected
  point P0 (0, 0)
  dimension "d47" = 2.8
  dimension "d48" = 2.8
  dimension "d49" = 2.8
  dimension "d50" = 2.8
  constraints: 4 centre point
  measures "d47" diameter of A0
  measures "d48" diameter of A1
  measures "d49" diameter of A2
  measures "d50" diameter of A3
extrude "Extrusion5" cut sketch "Skizze7" against normal blind 10 contours A4 | A5 | A6 | A7 | A8 | A9 | A10 | A11
sketch "Skizze8" plane through (-11.5959, -57.9, 4) normal (0, -1, 0) x (1, 0, 0)
  circle A0 centre (105.5, -19.0756) radius 0.9 projected
  circle A1 centre (105.5, -40.1278) radius 0.9 projected
  line L0 (103, -47.0289) -> (103, -14) projected
  line L1 (103, -47.0289) -> (108, -47.0289) projected
  line L2 (108, -14) -> (108, -47.0289) projected
  line L3 (103, -14) -> (108, -14) projected
  line L4 (109, 0) -> (109, -68.1) projected
  line L5 (0, 0) -> (109, 0) projected
  line L6 (0, -68.1) -> (0, 0) projected
  arc A2 (99, -53.1) -> (103, -49.1) centre (99, -49.1) ccw projected
  line L7 (99, -53.1) -> (10, -53.1) projected
  arc A3 (6, -49.1) -> (10, -53.1) centre (10, -49.1) ccw projected
  line L8 (6, -49.1) -> (6, -14) projected
  arc A4 (10, -10) -> (6, -14) centre (10, -14) ccw projected
  line L9 (10, -10) -> (99, -10) projected
  arc A5 (103, -14) -> (99, -10) centre (99, -14) ccw projected
  line L10 (103, -14) -> (103, -49.1) projected
  circle A6 centre (3.5, -40.1278) radius 0.9
  circle A7 centre (3.5, -14) radius 0.9
  line L11 (109, -68.1) -> (0, -68.1) projected
  point P0 (11.5959, -4)
  dimension "d41" = 1.8
  dimension "d42" = 1.8
  dimension "d43" = 2.5
  dimension "d44" = 2.5
  constraints: 2 centre point
  measures "d41" diameter of A6
  measures "d42" diameter of A7
  measures "d43" distance from line of A6.centre L8
  measures "d44" distance from line of L8 A7.centre
extrude "Extrusion6" cut sketch "Skizze8" against normal blind 10 contours A0 | A1 | A6 | A7
sketch "Sketch9" plane through (0, 0, 4) normal (0, 0, 1) x (1, 0, 0)
  arc A0 (97.4041, -57.9) -> (101.4041, -53.9) centre (97.4041, -53.9) ccw projected
  line L0 (101.4041, -53.9) -> (101.4041, 18.1) projected
  arc A1 (101.4041, 18.1) -> (97.4041, 22.1) centre (97.4041, 18.1) ccw projected
  line L1 (97.4041, 22.1) -> (-11.5959, 22.1) projected
  arc A2 (-11.5959, 22.1) -> (-15.5959, 18.1) centre (-11.5959, 18.1) ccw projected
  line L2 (-15.5959, 18.1) -> (-15.5959, -53.9) projected
  arc A3 (-15.5959, -53.9) -> (-11.5959, -57.9) centre (-11.5959, -53.9) ccw projected
  line L3 (-11.5959, -57.9) -> (97.4041, -57.9) projected
  point P0 (0, 0)
extrude "Extrusion7" cut sketch "Sketch9" against normal blind 4
ref_plane "Work Plane5" through (42.9041, -53.9, -64.1) normal (-1, 0, 0) x (0, 0, 1)
ref_plane "Work Plane6" through (-11.5959, -17.9, -64.1) normal (0, -1, 0) x (1, 0, 0)
sketch "Sketch10" plane through (101.4041, -53.9, -64.1) normal (1, 0, 0) x (0, 0, -1)
  circle A0 centre (-4, 1.1654) radius 0.5 projected
  circle A1 centre (-24, 1.1654) radius 0.5 projected
  line L0 (-13, 3) -> (-13, 9) projected
  line L1 (-13, 9) -> (-14, 9) projected
  line L2 (-14, 9) -> (-14, 3) projected
  line L3 (-14, 3) -> (-26, 3) projected
  line L4 (-26, 3) -> (-26, -3) projected
  line L5 (-26, -3) -> (-20.5, -3) projected
  line L6 (-20.5, -7.4105) -> (-20.5, -9) projected
  line L7 (-20.5, -9) -> (-6.5, -9) projected
  line L8 (-6.5, -3) -> (-1, -3) projected
  line L9 (-1, -3) -> (-1, 3) projected
  line L10 (-1, 3) -> (-13, 3) projected
  circle A2 centre (-24, -5.4346) radius 0.5 projected
  line L11 (-20.5, -4.0361) -> (-26, -4.0361) projected
  line L12 (-26, -4.0361) -> (-26, -7.4105) projected
  line L13 (-26, -7.4105) -> (-20.5, -7.4105) projected
  line L14 (-6.5, -9) -> (-6.5, -3) projected
  line L15 (-20.5, -3) -> (-20.5, -4.0361) projected
  point P0 (-64.1, 53.9)
extrude "Extrusion8" cut sketch "Sketch10" against normal blind 10 contours A0 | A1
equation "\"d59\" = 0.5 * d58"
equation "\"d61\" = 0.5 * d60"
